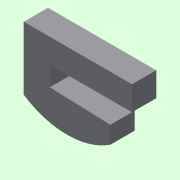
# Autodesk Inventor part: Cuvette_retainer2
Saved by Autodesk Inventor 2015 (Build 190159000, 159)
## iProperties
Created: 2015-06-21
Part Number: Cuvette_retainer2
Material: Generic
Document SubType Name: Modeling
Designer: Openlab
Density: 1 g/cm^3
Appearance: Default
Author: Openlab
Autodesk Inventor part; units mm, degrees
ref_plane "YZ Plane" through (0, 0, 0) normal (1, 0, 0) x (0, 1, 0)
ref_plane "XZ Plane" through (0, 0, 0) normal (0, 1, 0) x (-1, 0, 0)
ref_plane "XY Plane" through (0, 0, 0) normal (0, 0, 1) x (1, 0, 0)
sketch "Sketch1" plane through (0, 0, 0) normal (0, 1, 0) x (-1, 0, 0)
  line L0 (0, 0) -> (0, -2.8)
  line L1 (0, -2.8) -> (9.5, -2.8)
  line L2 (0, 0) -> (12.5, 0)
  line L3 (12.5, 0) -> (12.5, -2.8)
  line L4 (9.5, -2.8) -> (9.5, -5.05)
  line L5 (9.5, -5.05) -> (2.5, -5.3)
  line L6 (2.5, -5.3) -> (2.5, -7.3)
  line L7 (12.5, -7.3) -> (12.5, -7.3)
  line L8 (12.5, -7.3) -> (12.5, -2.8)
  line L9 (12.5, -2.8) -> (12.5, -2.8)
  arc A0 (2.5, -7.3) -> (12.5, -7.3) centre (7.5, 0.2833) ccw
  line L10 (14.5304, -7.3) -> (10.3082, -7.3) construction
  dimension "d1" = 2.8
  dimension "d2" = 12.5
  dimension "d3" = 9.5
  dimension "d4" = 3
  dimension "d6" = 4.5
  dimension "d8" = 7.5
  dimension "d9" = 2
  dimension "d13" = 2.25
  dimension "d14" = 10
  dimension "d15" = 1.5
  constraints: 22 end point, 5 perpendicular, 3 point on line, 2 horizontal, 2 point on circle, 2 vertical, 1 centre point
  measures "d1" distance of L0.start L0.end
  measures "d2" distance of L0.start L2.end
  measures "d3" distance of L0.end L1.end
  measures "d4" distance between parallel lines of L4 L8
  measures "d6" distance of L7.end L8.end
  measures "d8" distance from line of L0 A0.centre
  measures "d9" distance of L5.end L6.end
  measures "d13" distance of L1.end L4.end
  measures "d14" distance from line of L6 L7.start
  measures "d15" distance edge to line of A0 L10
extrude "Extrusion1" add sketch "Sketch1" along normal blind 2.8
body "Solid1"
